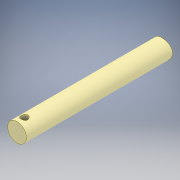
# Autodesk Inventor part: Ground_Antenna700mm_SupportArm
Saved by Autodesk Inventor 2018 (Build 220112000, 112)
## iProperties
Created: 2018-10-12
Part Number: Ground_Antenna700mm_SupportArm
Material: Nylon 6/6
Document SubType Name: Modeling
Designer: Bradley
Density: 1.13 g/cm^3
Appearance: Nylon 6
Mass: 3.45513 g
Surface Area: 14.4305 cm^2
Volume: 3.05764 cm^3
Author: Bradley
Autodesk Inventor part; units mm, degrees
ref_plane "YZ Plane" through (0, 0, 0) normal (1, 0, 0) x (0, 1, 0)
ref_plane "XZ Plane" through (0, 0, 0) normal (0, 1, 0) x (-1, 0, 0)
ref_plane "XY Plane" through (0, 0, 0) normal (0, 0, 1) x (1, 0, 0)
sketch "Sketch2" plane through (0, 0, 0) normal (0, 1, 0) x (-1, 0, 0)
  circle A0 centre (0, 0) radius 6.35
  dimension "d10" = 12.7
  constraints: 1 centre point, 1 coincident
  measures "d10" diameter of A0
extrude "Extrusion2" add sketch "Sketch2" along normal mid plane 118.65
sketch "Sketch3" plane through (0, 0, 0) normal (0, 0, 1) x (1, 0, 0)
  line L0 (6.35, 59.325) -> (-6.35, 59.325) projected
  circle A0 centre (0, 59.325) radius 21.082
  line L1 (-6.35, -59.325) -> (6.35, -59.325) projected
  circle A1 centre (0, -54.325) radius 2.3813
  circle A2 centre (0, 59.325) radius 118.65
  line L2 (-6.35, -59.325) -> (-6.35, -59.155)
  line L3 (-6.35, -59.325) -> (-6.35, 59.325) projected
  line L4 (6.35, -59.325) -> (6.35, -59.155)
  line L5 (6.35, -59.325) -> (6.35, 59.325) projected
  point P0 (0, 0)
  dimension "d13" = 42.164
  dimension "d16" = 4.7625
  dimension "d17" = 5
  constraints: 4 end point, 3 centre point, 2 point on circle, 2 point on line, 1 coincident, 1 midpoint, 1 tangent, 1 vertical alignment
  measures "d13" diameter of A0
  measures "d16" diameter of A1
  measures "d17" distance from line of L1 A1.centre
extrude "Extrusion3" cut sketch "Sketch3" along normal through all both and the other way through all contours L5 A0 L3 L0 | L0 L3 A0 L5 | L4 L1 A2 | A2 L1 L2 | A1
body "Solid2"
